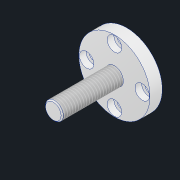
# Autodesk Inventor part: adapter1
Saved by Autodesk Inventor 2022 (Build 260153000, 153)
## iProperties
Created: 2021-11-12
Part Number: adapter1
Material: アルミニウム 6061
Document SubType Name: Modeling
Designer: Yuta Kage
Density: 2.7 g/cm^3
Appearance: アルミニウム - フラット
Author: Yuta Kage
Autodesk Inventor part; units mm, degrees
ref_plane "YZ Plane" through (0, 0, 0) normal (1, 0, 0) x (0, 1, 0)
ref_plane "XZ Plane" through (0, 0, 0) normal (0, 1, 0) x (-1, 0, 0)
ref_plane "XY Plane" through (0, 0, 0) normal (0, 0, 1) x (1, 0, 0)
sketch "スケッチ1" plane through (0, 0, 0) normal (1, 0, 0) x (0, 1, 0)
  line L0 (0, 33) -> (4, 33)
  line L1 (4, 33) -> (4, 5.5)
  line L2 (4, 5.5) -> (16, 5.5)
  line L3 (16, 5.5) -> (16, 0)
  line L4 (0, 33) -> (0, 2.5)
  line L5 (0, 2.5) -> (6, 2.5)
  line L6 (6, 2.5) -> (6, 0)
  line L7 (6, 0) -> (16, 0)
  point P0 (0, 0)
  dimension "d0" = 4
  dimension "d2" = 5.5
  dimension "d3" = 27.5
  dimension "d22" = 2.5
  dimension "d23" = 6
  dimension "d24" = 16
  constraints: 16 end point, 6 perpendicular, 2 point on line, 1 horizontal, 1 vertical
  measures "d0" distance of L0.start L0.end
  measures "d2" distance of L2.end L3.end
  measures "d3" distance of L0.end L1.end
  measures "d22" distance of L5.end L6.end
  measures "d23" distance of L4.end L5.end
  measures "d24" distance between parallel lines of L3 L4
revolve "回転1" add sketch "スケッチ1" angle 360 about axis through (0, 0, 33) along (0, 0, -1)
sketch "スケッチ2" plane through (0, 0, 5.5) normal (0, 0, 1) x (1, 0, 0)
  circle A0 centre (0, 0) radius 12.5
  point P0 (0, 0)
  point P1 (0, 12.5)
  point P2 (-12.5, 0)
  point P3 (0, -12.5)
  point P4 (12.5, 0)
  dimension "d5" = 25
  dimension "d8" = 360
  constraints: 1 coincident, 1 vertical alignment, 7 other
hole "穴1" at (0, 12.5, 5.5) at (-12.5, 0, 5.5) at (0, -12.5, 5.5) at (12.5, 0, 5.5) direction (0, 0, -1) diameter 3.4 end through all counterbore diameter 6.5 counterbore depth 3 clearance for "Socket Head Cap Screw" size "M3" standard "Ansi Metric M Profile"
thread "ねじ1" size "M8x1.25" class "6g" standard "ANSI Metric M Profile" full length
chamfer "面取り1" distance 0.5 angle 45 1 edges at (0, -4, 33)
